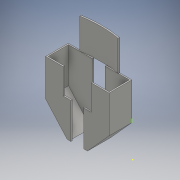
# Autodesk Inventor part: full gear cad
Saved by Autodesk Inventor 2016 (Build 200138000, 138)
## iProperties
Created: 2017-01-21
Part Number: full gear cad
Material: Generic
Document SubType Name: Modeling
Designer: decoteaub
Density: 1 g/cm^3
Appearance: Default
Author: decoteaub
Autodesk Inventor part; units mm, degrees
ref_plane "YZ Plane" through (0, 0, 0) normal (1, 0, 0) x (0, 1, 0)
ref_plane "XZ Plane" through (0, 0, 0) normal (0, 1, 0) x (-1, 0, 0)
ref_plane "XY Plane" through (0, 0, 0) normal (0, 0, 1) x (1, 0, 0)
sketch "Sketch1" plane through (0, 0, 0) normal (0, 0, 1) x (1, 0, 0)
  line L0 (9.560424, 344.540635) -> (9.560424, 166.740635)
  line L1 (9.560424, 166.740635) -> (123.860424, 39.740635)
  line L2 (123.860424, 39.740635) -> (130.210424, 39.740635)
  line L3 (130.210424, 39.740635) -> (130.210424, 217.540635)
  line L4 (130.210424, 217.540635) -> (92.110424, 217.540635)
  line L5 (92.110424, 217.540635) -> (92.110424, 344.540635)
  line L6 (92.110424, 344.540635) -> (9.560424, 344.540635)
  line L7 (193.710424, 217.540635) -> (193.710424, 39.740635)
  line L8 (193.710424, 39.740635) -> (200.060424, 39.740635)
  line L9 (200.060424, 39.740635) -> (314.360424, 166.740635)
  line L10 (314.360424, 166.740635) -> (314.360424, 344.540635)
  line L11 (314.360424, 344.540635) -> (231.810424, 344.540635)
  line L12 (231.810424, 344.540635) -> (231.810424, 217.540635)
  line L13 (231.810424, 217.540635) -> (193.710424, 217.540635)
  point P0 (0, 0)
  dimension "d0" = 127
  dimension "d1" = 38.1
  dimension "d2" = 177.8
  dimension "d3" = 127
  dimension "d4" = 82.55
  dimension "d5" = 6.35
  dimension "d9" = 63.5
  dimension "d10" = 38.1
  dimension "d11" = 82.55
  dimension "d12" = 6.35
  dimension "d13" = 177.8
  dimension "d14" = 170.86103
  dimension "d15" = 127
  dimension "d16" = 177.8
  constraints: 28 end point, 8 perpendicular, 3 vertical, 1 parallel
  measures "d0" distance of L4.end L5.end
  measures "d1" distance of L3.end L4.end
  measures "d2" distance of L0.start L0.end
  measures "d3" vertical distance of L0.end L1.end
  measures "d4" distance of L5.end L0.start
  measures "d5" distance of L1.end L2.end
  measures "d9" distance between parallel lines of L7 L3
  measures "d10" distance of L12.end L7.start
  measures "d11" distance of L10.end L11.end
  measures "d12" distance of L7.end L8.end
  measures "d13" distance of L7.start L7.end
  measures "d14" distance of L8.end L9.end
  measures "d15" distance of L11.end L12.end
  measures "d16" distance of L9.end L10.end
extrude "Extrusion1" add sketch "Sketch1" along normal blind 6.35
sketch "Sketch2" plane through (0, 0, 6.35) normal (0, 0, 1) x (1, 0, 0)
  line L0 (9.560424, 166.740635) -> (123.860424, 39.740635)
  line L1 (9.560424, 166.740635) -> (123.860424, 39.740635)
  line L2 (123.860424, 39.740635) -> (116.804868, 33.390635)
  line L3 (116.804868, 33.390635) -> (2.504868, 160.390635)
  line L4 (2.504868, 160.390635) -> (9.560424, 166.740635)
  line L5 (314.360424, 166.740635) -> (201.350031, 39.740635)
  line L6 (201.350031, 39.740635) -> (207.700031, 34.090115)
  line L7 (207.700031, 34.090115) -> (320.710424, 161.090115)
  line L8 (320.710424, 161.090115) -> (314.360424, 166.740635)
  line L9 (9.560424, 166.740635) -> (3.210424, 166.740635)
  line L10 (3.210424, 166.740635) -> (3.210424, 369.270371)
  line L11 (3.210424, 369.270371) -> (9.560424, 369.270371)
  line L12 (9.560424, 369.270371) -> (9.560424, 166.740635)
  line L13 (314.360424, 166.740635) -> (314.360424, 344.540635)
  line L14 (314.360424, 344.540635) -> (320.710424, 344.540635)
  line L15 (320.710424, 344.540635) -> (320.710424, 141.340635)
  line L16 (320.710424, 141.340635) -> (314.360424, 141.340635)
  line L17 (314.360424, 141.340635) -> (314.360424, 344.540635)
  point P0 (0, 0)
  dimension "d17" = 6.35
  dimension "d18" = 6.35
  dimension "d19" = 6.35
  dimension "d20" = 6.35
  constraints: 32 end point, 8 perpendicular, 5 equal length, 2 horizontal
  measures "d17" vertical distance of L3.end L0.start
  measures "d18" horizontal distance of L5.end L6.end
  measures "d19" distance of L13.end L14.end
  measures "d20" distance of L10.end L11.end
sketch "Sketch2 outline for Extrusion2" plane through (0, 0, 6.35) normal (0, 0, 1) x (1, 0, 0)
  line L0 (3.210424, 166.740635) -> (9.560424, 166.740635)
  line L1 (3.210424, 369.270371) -> (3.210424, 166.740635)
  line L2 (9.560424, 369.270371) -> (3.210424, 369.270371)
  line L3 (9.560424, 166.740635) -> (9.560424, 369.270371)
  line L4 (320.710424, 344.540635) -> (314.360424, 344.540635)
  line L5 (314.360424, 344.540635) -> (314.360424, 166.740635)
  line L6 (314.360424, 166.740635) -> (201.350031, 39.740635)
  line L7 (201.350031, 39.740635) -> (207.700031, 34.090115)
  line L8 (207.700031, 34.090115) -> (314.360424, 153.954046)
  line L9 (314.360424, 153.954046) -> (314.360424, 141.340635)
  line L10 (314.360424, 141.340635) -> (320.710424, 141.340635)
  line L11 (320.710424, 141.340635) -> (320.710424, 344.540635)
  line L12 (123.860424, 39.740635) -> (9.560424, 166.740635)
  line L13 (116.804868, 33.390635) -> (123.860424, 39.740635)
  line L14 (2.504868, 160.390635) -> (116.804868, 33.390635)
  line L15 (9.560424, 166.740635) -> (2.504868, 160.390635)
extrude "Extrusion2" add sketch "Sketch2 outline for Extrusion2" along normal blind 101.6
sketch "Sketch4" plane through (0, 0, 0) normal (0, 0, -1) x (-1, 0, 0)
  line L0 (-193.710424, 39.740635) -> (-200.060424, 39.740635)
  line L1 (-193.710424, 39.740635) -> (-216.217025, 39.740635)
  line L2 (-216.217025, 39.740635) -> (-216.217025, 32.649574)
  line L3 (-216.217025, 32.649574) -> (-193.710424, 32.649574)
  line L4 (-193.710424, 32.649574) -> (-193.710424, 39.740635)
  line L5 (-123.860424, 39.740635) -> (-130.210424, 39.740635)
  line L6 (-130.210424, 39.740635) -> (-108.923155, 39.740635)
  line L7 (-108.923155, 39.740635) -> (-108.923155, 31.510409)
  line L8 (-108.923155, 31.510409) -> (-130.210424, 31.510409)
  line L9 (-130.210424, 31.510409) -> (-130.210424, 39.740635)
  point P0 (0, 0)
  point P1 (-200.060424, 14.340635)
  point P2 (-123.860424, 14.340635)
  constraints: 16 end point, 4 parallel, 2 horizontal, 2 perpendicular, 2 other
extrude "Extrusion4" cut sketch "Sketch4" against normal blind 114.3
sketch "Sketch5" plane through (0, 0, 107.95) normal (0, 0, 1) x (1, 0, 0)
  line L0 (3.210424, 141.340635) -> (3.210424, 343.870371)
  line L1 (3.210424, 343.870371) -> (130.210424, 343.870371)
  line L2 (92.110424, 344.540635) -> (9.560424, 344.540635)
  line L3 (130.210424, 39.740635) -> (130.210424, 217.540635)
  line L4 (130.210424, 343.870371) -> (130.210424, 39.740635)
  line L5 (123.860424, 39.740635) -> (130.210424, 39.740635)
  line L6 (130.210424, 14.340635) -> (111.089868, 14.340635)
  line L7 (111.089868, 14.340635) -> (2.504868, 134.990635)
  line L8 (111.089868, 14.340635) -> (2.504868, 134.990635)
  line L9 (2.504868, 134.990635) -> (3.210424, 141.340635)
  line L10 (193.710424, 39.740635) -> (193.710424, 344.540635)
  line L11 (193.710424, 344.540635) -> (320.710424, 344.540635)
  line L12 (320.710424, 141.340635) -> (320.710424, 344.540635)
  line L13 (320.710424, 344.540635) -> (320.710424, 141.340635)
  line L14 (314.360424, 344.540635) -> (314.360424, 141.340635)
  line L15 (320.710424, 135.690115) -> (314.360424, 141.340635)
  line L16 (320.710424, 141.340635) -> (320.710424, 135.690115)
  line L17 (320.710424, 135.690115) -> (235.3302, 39.740635)
  line L18 (235.3302, 39.740635) -> (193.710424, 39.740635)
  point P0 (0, 0)
  constraints: 22 end point, 3 collinear, 3 parallel, 2 perpendicular, 1 horizontal, 1 vertical, 1 other
sketch "Sketch5 outline for Extrusion5" plane through (0, 0, 107.95) normal (0, 0, 1) x (1, 0, 0)
  line L0 (193.710424, 344.540635) -> (193.710424, 39.740635)
  line L1 (193.710424, 39.740635) -> (235.3302, 39.740635)
  line L2 (235.3302, 39.740635) -> (320.710424, 135.690115)
  line L3 (320.710424, 135.690115) -> (320.710424, 344.540635)
  line L4 (320.710424, 344.540635) -> (193.710424, 344.540635)
  line L5 (3.210424, 343.870371) -> (3.210424, 141.340635)
  line L6 (130.210424, 343.870371) -> (3.210424, 343.870371)
  line L7 (130.210424, 39.740635) -> (130.210424, 343.870371)
  line L8 (111.089868, 14.340635) -> (130.210424, 39.740635)
  line L9 (2.504868, 134.990635) -> (111.089868, 14.340635)
  line L10 (3.210424, 141.340635) -> (2.504868, 134.990635)
extrude "Extrusion5" add sketch "Sketch5 outline for Extrusion5" along normal blind 6.35
sketch "Sketch6" plane through (193.710424, 39.740635, 107.95) normal (-1, 0, 0) x (0, 0, 1)
  line L0 (0, 304.8) -> (0, 0) projected
  line L1 (6.35, 0) -> (-101.6, 0) projected
  line L2 (0, 101.6) -> (6.35, 101.6)
  line L3 (6.35, 101.6) -> (6.35, 0)
  line L4 (6.35, 0) -> (0, 0)
  line L5 (0, 0) -> (0, 101.6)
  point P0 (-107.95, -39.740635)
  point P1 (-107.95, 0)
  dimension "d29" = 101.6
  constraints: 8 end point, 2 parallel, 1 horizontal, 1 perpendicular, 1 point on line
  measures "d29" distance of L2.end L1.start
extrude "Extrusion6" add sketch "Sketch6" along normal blind 63.5
sketch "Sketch7" plane through (0, 0, 0) normal (0, 0, -1) x (-1, 0, 0)
  line L0 (-3.210424, 343.870371) -> (-3.210424, 141.340635)
  line L1 (-3.210424, 147.802494) -> (-9.560424, 147.802494)
  line L2 (-9.560424, 147.802494) -> (-9.560424, 134.679374)
  line L3 (-9.560424, 134.679374) -> (-3.210424, 134.679374)
  line L4 (-3.210424, 134.679374) -> (-3.210424, 147.802494)
  line L5 (-314.360424, 166.740635) -> (-201.350031, 39.740635)
  line L6 (-320.714268, 135.664797) -> (-320.714268, 145.552556)
  line L7 (-320.738877, 135.664797) -> (-314.360424, 135.664797)
  line L8 (-314.360424, 135.664797) -> (-314.360424, 145.552556)
  line L9 (-314.360424, 166.740635) -> (-314.360424, 344.540635)
  line L10 (-320.714268, 145.552556) -> (-314.360424, 145.552556)
  line L11 (-320.738877, 135.664797) -> (-314.360424, 135.664797)
  line L12 (-314.360424, 135.664797) -> (-314.360424, 145.552556)
  line L13 (-314.360424, 145.552556) -> (-320.738877, 145.552556)
  line L14 (-320.738877, 145.552556) -> (-320.738877, 135.664797)
  point P0 (0, 0)
  point P1 (-309.309804, 161.064797)
  point P2 (-314.360424, 141.340635)
  point P3 (-201.350031, 39.740635)
  constraints: 24 end point, 4 parallel, 3 horizontal, 3 perpendicular, 2 point on line, 2 other
sketch "Sketch8" plane through (0, 0, 0) normal (0, 0, -1) x (-1, 0, 0)
  line L0 (-3.210424, 141.340635) -> (-3.210424, 343.870371)
  line L1 (-3.210424, 141.825243) -> (-1.362602, 141.825243)
  line L2 (-1.362602, 141.825243) -> (-1.362602, 134.146464)
  line L3 (-1.362602, 134.146464) -> (-3.210424, 134.146464)
  line L4 (-3.210424, 134.146464) -> (-3.210424, 141.825243)
  point P0 (0, 0)
  point P1 (-3.210424, 135.625635)
  constraints: 8 end point, 2 parallel, 1 horizontal, 1 perpendicular, 1 point on line
extrude "Extrusion8" cut sketch "Sketch8" against normal blind 114.3
sketch "Sketch10" plane through (231.810424, 344.540635, 0) normal (0, 1, 0) x (1, 0, 0)
  line L0 (88.9, -114.3) -> (-38.1, -114.3)
  line L1 (-101.6, -114.3) -> (-228.6, -114.3)
  line L2 (-101.6, -107.95) -> (-222.25, -107.95)
  line L3 (82.55, -107.95) -> (-30.460392, -107.95)
  arc A0 (-165.1, -107.95) -> (25.4, -107.95) centre (-69.85, 433.719551) ccw
  line L4 (88.9, -6.35) -> (88.9, -114.3)
  line L5 (-228.6, -107.95) -> (-228.6, -114.3)
  line L6 (-165.1, -107.95) -> (-167.602477, -114.3)
  line L7 (25.4, -107.95) -> (28.412743, -114.3)
  line L8 (3.519776, -114.3) -> (88.9, -114.3)
  arc A1 (-167.602477, -114.3) -> (28.412743, -114.3) centre (-69.594867, 400.309912) ccw
  point P0 (-231.810424, 0)
  point P1 (-165.1, -114.3)
  point P2 (25.4, -114.3)
  point P3 (77.518866, -107.95)
  point P4 (88.9, 0)
  point P5 (-228.6, 0)
  point P6 (88.896956, -114.3)
  dimension "d38" = 190.5
  dimension "d39" = 63.5
  dimension "d40" = 63.5
  dimension "d44" = 63.5
  dimension "d45" = 63.5
  constraints: 4 end point, 4 point on circle, 4 point on line, 2 centre point, 2 midpoint
  measures "d38" distance of point (-165.1, -114.3) point (25.4, -114.3)
  measures "d39" distance of L0.start point (25.4, -114.3)
  measures "d40" distance of L1.end point (-165.1, -114.3)
  measures "d44" distance from line of L4 L7.start
  measures "d45" distance from line of L5 L6.start
extrude "Extrusion10" add sketch "Sketch10" along normal blind 152.4
extrude "Extrusion11" add sketch "Sketch7" against normal blind 114.3
sketch "Sketch11" plane through (193.710424, 141.340635, 114.3) normal (0, 1, 0) x (1, 0, 0)
  line L0 (0, 6.35) -> (0, 0)
  line L1 (-63.505152, 0) -> (0, 0)
  line L2 (0, 0) -> (0, 6.35)
  line L3 (0, 6.35) -> (-63.505152, 6.35)
  line L4 (-63.505152, 6.35) -> (-63.505152, 0)
  line L5 (0, 0) -> (-63.5, 0)
  point P0 (-193.710424, 114.3)
  constraints: 8 end point, 2 parallel, 1 collinear, 1 horizontal, 1 perpendicular
extrude "Extrusion12" add sketch "Sketch11" along normal blind 25.4
sketch "Sketch12" plane through (0, 0, 107.95) normal (0, 0, 1) x (1, 0, 0)
  line L0 (130.210424, 343.870371) -> (9.560424, 343.870371)
  line L1 (3.210424, 369.270371) -> (3.210424, 166.740635)
  line L2 (9.560424, 343.870371) -> (3.210424, 343.870371)
  line L3 (3.210424, 343.870371) -> (3.210424, 369.270371)
  line L4 (3.210424, 369.270371) -> (9.560424, 369.270371)
  line L5 (9.560424, 369.270371) -> (9.560424, 343.870371)
  point P0 (0, 0)
  constraints: 8 end point, 2 parallel, 1 horizontal, 1 perpendicular
extrude "Extrusion13" cut sketch "Sketch12" against normal blind 114.3
sketch "Sketch13" plane through (3.210424, 166.740635, 6.35) normal (-1, 0, 0) x (0, 0, 1)
  line L0 (107.95, -32.533951) -> (107.95, -152.4)
  line L1 (-6.35, -18.909661) -> (107.95, -18.909661)
  line L2 (107.95, -18.909661) -> (107.95, -32.533951)
  line L3 (107.95, -32.533951) -> (-6.35, -32.533951)
  line L4 (-6.35, -32.533951) -> (-6.35, -18.909661)
  line L5 (101.6, -127) -> (101.6, 0)
  line L6 (101.6, 0) -> (107.95, 0)
  line L7 (107.95, 0) -> (107.95, -18.909661)
  line L8 (107.95, -18.909661) -> (101.6, -18.909661)
  line L9 (101.6, -18.909661) -> (101.6, 0)
  point P0 (-6.35, -166.740635)
  constraints: 16 end point, 4 parallel, 2 horizontal, 2 perpendicular
extrude "Extrusion14" cut sketch "Sketch13" against normal blind 6.35
sketch "Sketch14" plane through (0, 0, 107.95) normal (0, 0, -1) x (-1, 0, 0)
  line L0 (-9.560424, 152.551129) -> (-9.560424, 166.740635)
  line L1 (-9.560424, 134.206684) -> (-3.210424, 134.206684)
  line L2 (-9.560424, 152.551129) -> (-9.560424, 134.206684)
  line L3 (-9.560424, 134.206684) -> (-3.210424, 134.206684)
  line L4 (-3.210424, 134.206684) -> (-111.089868, 14.340635)
  line L5 (-3.210424, 134.206684) -> (-111.089868, 14.340635)
  line L6 (-111.089868, 14.340635) -> (-130.210424, 39.740635)
  line L7 (-111.089868, 14.340635) -> (-130.210424, 39.740635)
  line L8 (-111.089868, 39.740635) -> (-123.860424, 39.740635)
  line L9 (-130.210424, 39.740635) -> (-111.089868, 39.740635)
  line L10 (-111.089868, 39.740635) -> (-9.560424, 152.551129)
  point P0 (0, 0)
  constraints: 12 end point, 4 collinear, 1 parallel, 1 point on line, 1 vertical
extrude "Extrusion15" cut sketch "Sketch14" against normal blind 6.35
sketch "Sketch16" plane through (0, 0, 107.95) normal (0, 0, -1) x (-1, 0, 0)
  line L0 (-314.360424, 153.954046) -> (-314.360424, 145.552556)
  line L1 (-314.360424, 135.664797) -> (-314.360424, 145.552556)
  line L2 (-314.360424, 153.954046) -> (-314.360424, 135.664797)
  line L3 (-320.738877, 135.664797) -> (-314.360424, 135.664797)
  line L4 (-314.360424, 135.664797) -> (-320.738877, 135.664797)
  line L5 (-235.3302, 39.740635) -> (-320.687894, 135.664797)
  line L6 (-320.738877, 135.664797) -> (-235.381183, 39.740635)
  line L7 (-212.728121, 39.740635) -> (-314.360424, 153.954046)
  line L8 (-235.381183, 39.740635) -> (-212.728121, 39.740635)
  line L9 (-212.728121, 39.740635) -> (-314.360424, 153.954046)
  point P0 (0, 0)
  constraints: 10 end point, 2 parallel, 1 collinear, 1 perpendicular, 1 vertical
extrude "Extrusion16" cut sketch "Sketch16" against normal blind 6.35
sketch "Sketch17" plane through (0, 0, 6.35) normal (0, 0, -1) x (-1, 0, 0)
  line L0 (-212.728121, 39.740635) -> (-314.360424, 153.954046)
  line L1 (-314.360424, 153.954046) -> (-320.710424, 160.522836)
  line L2 (-320.710424, 145.552556) -> (-320.710424, 344.540635)
  line L3 (-320.710424, 145.552556) -> (-314.360424, 145.552556)
  line L4 (-320.710424, 145.552556) -> (-314.360424, 145.552556)
  line L5 (-314.360424, 145.552556) -> (-314.360424, 153.954046)
  line L6 (-314.360424, 153.954046) -> (-314.360424, 135.664797)
  line L7 (-314.360424, 145.552556) -> (-320.710424, 145.552556)
  line L8 (-320.710424, 145.552556) -> (-320.710424, 153.954046)
  line L9 (-320.710424, 153.954046) -> (-314.360424, 153.954046)
  line L10 (-314.360424, 153.954046) -> (-314.360424, 145.552556)
  line L11 (-320.710424, 160.522836) -> (-314.360424, 153.954046)
  line L12 (-320.710424, 160.522836) -> (-320.710424, 153.954046)
  point P0 (0, 0)
  constraints: 18 end point, 3 collinear, 3 point on line, 2 parallel, 1 horizontal, 1 perpendicular
extrude "Extrusion17" cut sketch "Sketch17" against normal blind 152.4
sketch "Sketch18" plane through (0, 0, 0) normal (0, 0, -1) x (-1, 0, 0)
  line L0 (-314.360424, 145.552556) -> (-320.738877, 145.552556)
  line L1 (-320.738877, 145.552556) -> (-314.360424, 145.552556)
  line L2 (-314.360424, 145.552556) -> (-314.360424, 135.51)
  line L3 (-314.360424, 135.51) -> (-320.738877, 135.51)
  line L4 (-320.738877, 135.51) -> (-320.738877, 145.552556)
  point P0 (0, 0)
  constraints: 8 end point, 2 parallel, 1 horizontal, 1 perpendicular
extrude "Extrusion18" cut sketch "Sketch18" against normal blind 152.4
sketch "Sketch19" plane through (0, 0, 6.35) normal (0, 0, -1) x (-1, 0, 0)
  line L0 (-111.089868, 39.740635) -> (-212.728121, 39.740635)
  line L1 (-124.141437, 39.740635) -> (-111.089868, 39.740635)
  line L2 (-9.560424, 343.870371) -> (-9.560424, 166.740635)
  line L3 (-9.560424, 343.870371) -> (-3.073851, 343.870371)
  line L4 (-3.073851, 343.870371) -> (-3.073851, 166.740635)
  line L5 (-3.073851, 166.740635) -> (-9.560424, 166.740635)
  line L6 (-9.560424, 166.740635) -> (-9.560424, 343.870371)
  line L7 (-314.360424, 166.740635) -> (-314.360424, 344.540635)
  line L8 (-314.360424, 153.954046) -> (-320.710424, 160.522836)
  line L9 (-314.360424, 344.540635) -> (-320.710424, 344.540635)
  line L10 (-320.710424, 344.540635) -> (-320.710424, 160.522836)
  line L11 (-320.710424, 160.522836) -> (-314.360424, 160.522836)
  line L12 (-314.360424, 160.522836) -> (-314.360424, 344.540635)
  line L13 (-200.060424, 39.740635) -> (-314.360424, 166.740635)
  line L14 (-314.360424, 166.740635) -> (-314.360424, 160.522836)
  line L15 (-314.360424, 160.522836) -> (-320.710424, 160.522836)
  line L16 (-212.728121, 39.740635) -> (-314.360424, 153.954046)
  line L17 (-320.710424, 160.522836) -> (-320.710424, 344.540635)
  line L18 (-320.710424, 160.522836) -> (-212.728121, 39.740635)
  line L19 (-212.728121, 39.740635) -> (-200.060424, 39.740635)
  line L20 (-200.060424, 39.740635) -> (-314.360424, 166.740635)
  point P0 (0, 0)
  constraints: 28 end point, 4 parallel, 3 horizontal, 3 perpendicular, 1 point on line
extrude "Extrusion19" add sketch "Sketch19" along normal blind 6.35 contours L0 L16 L8 L11 L12 L13 | L12 L11 L10 L9 L7
sketch "Sketch20" plane through (0, 0, 6.35) normal (0, 0, -1) x (-1, 0, 0)
  line L0 (-9.560424, 166.740635) -> (-2.504868, 160.390635)
  line L1 (-9.560424, 160.390635) -> (-9.560424, 175.559995)
  line L2 (-3.210424, 343.870371) -> (-3.210424, 166.740635)
  line L3 (-9.560424, 166.740635) -> (-9.560424, 152.551129)
  line L4 (-3.210424, 176.563666) -> (-9.560424, 176.563666)
  line L5 (-9.560424, 176.563666) -> (-9.560424, 159.645882)
  line L6 (-9.560424, 159.645882) -> (-3.210424, 159.645882)
  line L7 (-3.210424, 159.645882) -> (-3.210424, 176.563666)
  point P0 (0, 0)
  constraints: 10 end point, 2 parallel, 1 horizontal, 1 midpoint, 1 perpendicular, 1 point on line
extrude "Extrusion20" add sketch "Sketch20" against normal blind 152.4
sketch "Sketch21" plane through (0, 0, 6.35) normal (0, 0, -1) x (-1, 0, 0)
  line L0 (-3.210424, 161.025635) -> (-2.504868, 160.390635)
  line L1 (-3.210424, 161.025635) -> (-2.32353, 161.025635)
  line L2 (-2.32353, 161.025635) -> (-2.32353, 159.41775)
  line L3 (-2.32353, 159.41775) -> (-3.210424, 159.41775)
  line L4 (-3.210424, 159.41775) -> (-3.210424, 161.025635)
  point P0 (0, 0)
  constraints: 8 end point, 2 parallel, 1 horizontal, 1 perpendicular
extrude "Extrusion21" cut sketch "Sketch21" against normal blind 152.4
sketch "Sketch22" plane through (3.210424, 176.563666, 114.3) normal (0, 1, 0) x (1, 0, 0)
  line L0 (0, 6.35) -> (0, -44.45)
  line L1 (0, -44.45) -> (6.35, -44.45)
  line L2 (0, 0.054609) -> (6.35, 0.054609)
  line L3 (6.35, 0.054609) -> (6.35, -44.45)
  line L4 (6.35, -44.45) -> (0, -44.45)
  line L5 (0, -44.45) -> (0, 0.054609)
  point P0 (-3.210424, 114.3)
  constraints: 8 end point, 2 parallel, 1 horizontal, 1 perpendicular, 1 point on line
extrude "Extrusion22" cut sketch "Sketch22" against normal blind 25.4
sketch "Sketch23" plane through (0, 0, 107.95) normal (0, 0, 1) x (1, 0, 0)
  line L0 (3.176222, 159.644687) -> (9.515247, 152.601326)
  line L1 (3.210424, 159.606684) -> (111.089868, 39.740635)
  line L2 (9.560424, 159.645882) -> (3.210424, 159.645882)
  line L3 (9.560424, 159.645882) -> (3.175146, 159.645882)
  line L4 (3.175146, 159.645882) -> (9.560424, 159.606684)
  line L5 (9.560424, 152.551129) -> (9.560424, 159.645882)
  line L6 (9.560424, 159.606684) -> (9.560424, 152.551129)
  line L7 (9.560424, 152.551129) -> (3.210424, 159.606684)
  line L8 (9.560424, 159.606684) -> (3.210424, 159.606684)
  line L9 (3.210424, 159.606684) -> (3.210424, 152.551129)
  line L10 (3.210424, 152.551129) -> (9.560424, 152.551129)
  line L11 (9.560424, 152.551129) -> (9.560424, 159.606684)
  point P0 (0, 0)
  constraints: 18 end point, 3 point on line, 2 collinear, 2 parallel, 1 horizontal, 1 perpendicular
extrude "Extrusion23" add sketch "Sketch23" along normal blind 6.35 contours L8 L5 L1 L0 | L0 L1 L10 L9
sketch "Sketch24" plane through (3.210424, 176.563666, 114.245391) normal (0, 0, 1) x (1, 0, 0)
  line L0 (6.35, 0) -> (6.35, -16.917784)
  line L1 (0, 0) -> (6.35, 0)
  line L2 (6.35, 0) -> (6.35, -16.917784)
  line L3 (6.35, -16.917784) -> (0, -16.917784)
  line L4 (0, -16.917784) -> (0, 0)
  point P0 (-3.210424, -176.563666)
  constraints: 8 end point, 2 parallel, 1 horizontal, 1 perpendicular
sketch "Sketch25" plane through (0, 0, 107.95) normal (0, 0, -1) x (-1, 0, 0)
  line L0 (-3.210424, 159.606684) -> (-111.089868, 39.740635)
  line L1 (-3.210424, 159.606684) -> (-9.560424, 152.551129)
  line L2 (-3.210424, 152.551129) -> (-9.560424, 152.551129)
  line L3 (-3.210424, 152.551129) -> (-3.210424, 159.606684)
  line L4 (-3.210424, 159.606684) -> (-3.210424, 152.551129)
  line L5 (-9.560424, 152.551129) -> (-3.210424, 152.551129)
  line L6 (-9.560424, 159.645882) -> (-3.210424, 159.645882)
  line L7 (-3.210424, 159.645882) -> (-9.560424, 152.551129)
  point P0 (0, 0)
  constraints: 8 end point, 3 point on line, 1 collinear
extrude "Extrusion24" cut sketch "Sketch25" against normal blind 25.4
sketch "Sketch26" plane through (0, 0, 6.35) normal (0, 0, -1) x (-1, 0, 0)
  line L0 (-123.860424, 39.740635) -> (-9.560424, 166.740635)
  line L1 (-111.089868, 39.740635) -> (-212.728121, 39.740635)
  line L2 (-123.860424, 39.740635) -> (-111.089868, 39.740635)
  line L3 (-3.210424, 159.606684) -> (-111.089868, 39.740635)
  line L4 (-111.089868, 39.740635) -> (-3.210424, 159.606684)
  line L5 (-3.210424, 159.606684) -> (-3.210424, 343.870371)
  line L6 (-3.210424, 159.606684) -> (-3.210424, 343.870371)
  line L7 (-3.210424, 343.870371) -> (-9.560424, 343.870371)
  line L8 (-130.210424, 343.870371) -> (-3.210424, 343.870371)
  line L9 (-9.560424, 344.540635) -> (-9.560424, 166.740635)
  line L10 (-9.560424, 166.740635) -> (-9.560424, 344.540635)
  line L11 (-3.210424, 159.606684) -> (-9.560424, 166.740635)
  line L12 (-9.560424, 166.740635) -> (-3.210424, 166.740635)
  point P0 (0, 0)
  constraints: 14 end point, 4 collinear, 2 point on line, 1 horizontal
sketch "Sketch26 outline for Extrusion25" plane through (0, 0, 6.35) normal (0, 0, -1) x (-1, 0, 0)
  line L0 (-9.560424, 166.740635) -> (-123.860424, 39.740635)
  line L1 (-123.860424, 39.740635) -> (-111.089868, 39.740635)
  line L2 (-111.089868, 39.740635) -> (-3.210424, 159.606684)
  line L3 (-3.210424, 159.606684) -> (-3.210424, 166.740635)
  line L4 (-3.210424, 166.740635) -> (-9.560424, 166.740635)
extrude "Extrusion25" add sketch "Sketch26 outline for Extrusion25" along normal blind 6.35
sketch "Sketch27" plane through (0, 0, 6.35) normal (0, 0, -1) x (-1, 0, 0)
  line L0 (-3.210424, 159.606684) -> (-3.210424, 166.740635)
  line L1 (-9.560424, 344.540635) -> (-9.560424, 166.740635)
  line L2 (-3.210424, 166.740635) -> (-9.560424, 166.740635)
  line L3 (-9.560424, 166.740635) -> (-9.560424, 344.540635)
  line L4 (-9.560424, 344.540635) -> (-3.210424, 344.540635)
  line L5 (-3.210424, 344.540635) -> (-3.210424, 166.740635)
  point P0 (0, 0)
  constraints: 8 end point, 2 parallel, 1 horizontal, 1 perpendicular
extrude "Extrusion26" add sketch "Sketch27" along normal blind 6.35
sketch "Sketch28" plane through (0, 0, 6.35) normal (0, 0, 1) x (1, 0, 0)
  line L0 (92.110424, 344.540635) -> (3.210424, 344.540635)
  line L1 (9.560424, 343.870371) -> (3.210424, 343.870371)
  line L2 (3.210424, 343.870371) -> (3.210424, 344.540635)
  line L3 (3.210424, 344.540635) -> (9.560424, 344.540635)
  line L4 (9.560424, 344.540635) -> (9.560424, 343.870371)
  point P0 (0, 0)
  constraints: 8 end point, 2 parallel, 1 horizontal, 1 perpendicular
extrude "Extrusion27" add sketch "Sketch28" along normal blind 107.95
sketch "Sketch29" plane through (9.560424, 166.740635, 6.35) normal (1, 0, 0) x (0, 0, -1)
  line L0 (-101.6, 0) -> (-101.6, 177.129736)
  line L1 (0, 177.8) -> (-107.95, 177.8)
  line L2 (-101.6, 177.129736) -> (-107.95, 177.129736)
  line L3 (-107.95, 177.129736) -> (-107.95, 177.8)
  line L4 (-107.95, 177.8) -> (-101.6, 177.8)
  line L5 (-101.6, 177.8) -> (-101.6, 177.129736)
  point P0 (6.35, -166.740635)
  constraints: 8 end point, 2 parallel, 1 horizontal, 1 perpendicular
extrude "Extrusion28" add sketch "Sketch29" along normal blind 57.15
sketch "Sketch30" plane through (9.560424, 166.740635, 6.35) normal (-1, 0, 0) x (0, 0, 1)
  line L0 (101.6, -7.094753) -> (107.895391, -7.094753)
  line L1 (101.6, -7.133951) -> (107.95, -7.133951)
  line L2 (101.6, -7.094753) -> (107.95, -7.094753)
  line L3 (107.95, -7.094753) -> (107.95, -7.133951)
  line L4 (107.95, -7.133951) -> (101.6, -7.133951)
  line L5 (101.6, -7.133951) -> (101.6, -7.094753)
  line L6 (107.895391, 9.823031) -> (107.95, 9.823031)
  line L7 (107.95, -7.094753) -> (107.895391, -7.094753)
  line L8 (107.895391, -7.094753) -> (107.895391, 9.823031)
  line L9 (107.895391, 9.823031) -> (107.95, 9.823031)
  line L10 (107.95, 9.823031) -> (107.95, -7.094753)
  point P0 (-6.35, -166.740635)
  constraints: 16 end point, 4 parallel, 2 horizontal, 2 perpendicular
extrude "Extrusion29" add sketch "Sketch30" along normal blind 6.35 contours L8 L6 L10 L2
body "Solid1"
